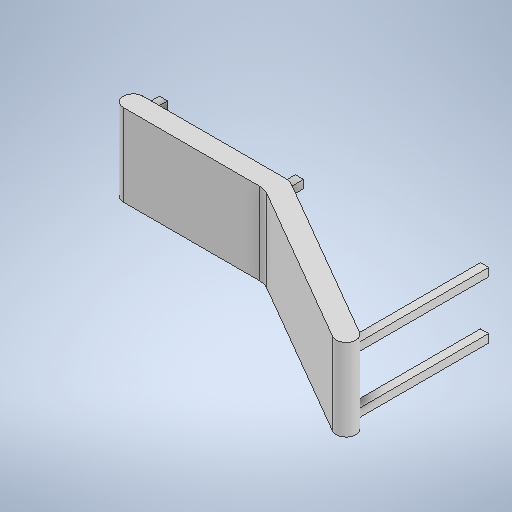
# Autodesk Inventor part: FirstConveyor
Saved by Autodesk Inventor 2025.1 (Build 291241000, 241)
## iProperties
Created: 2025-02-20
Part Number: FirstConveyor
Material: Generic
Document SubType Name: Modeling
Designer: yovan
Density: 1 g/cm^3
Appearance: Default
Author: yovan
Autodesk Inventor part; units mm, degrees
ref_plane "YZ Plane" through (0, 0, 0) normal (1, 0, 0) x (0, 1, 0)
ref_plane "XZ Plane" through (0, 0, 0) normal (0, 1, 0) x (-1, 0, 0)
ref_plane "XY Plane" through (0, 0, 0) normal (0, 0, 1) x (1, 0, 0)
sketch "Sketch1" plane through (0, 0, 0) normal (0, 1, 0) x (-1, 0, 0)
  line L0 (-60, 0) -> (-940, 0)
  line L1 (-891.5776, 120) -> (-60, 120)
  arc A0 (-60, 0) -> (-60, 120) centre (-60, 60) ccw
  line L2 (-60, 0) -> (-90, 0)
  arc A1 (-1909.8969, 691.9019) -> (-1970.1031, 588.0981) centre (-1940, 640) ccw
  line L3 (-1909.8969, 691.9019) -> (-951.7838, 136.1963)
  line L4 (-1970.1031, 588.0981) -> (-970.1031, 8.0981)
  arc A2 (-951.7838, 136.1963) -> (-891.5776, 120) centre (-891.5776, 240) ccw
  arc A3 (-970.1031, 8.0981) -> (-940, 0) centre (-940, 60) ccw
  line L5 (-60, 0) -> (-110, 0)
  line L6 (-110, 0) -> (-110, -100)
  line L7 (-110, -100) -> (-60, -100)
  line L8 (-60, -100) -> (-60, 0)
  line L9 (-940, 0) -> (-890, 0)
  line L10 (-890, 0) -> (-890, -100)
  line L11 (-890, -100) -> (-940, -100)
  line L12 (-940, -100) -> (-940, 0)
  line L13 (-1920.1031, 559.0981) -> (-1920.1031, -199.9999)
  line L14 (-1920.1031, -199.9999) -> (-1970.1031, -199.9999)
  line L15 (-1970.1031, -199.9999) -> (-1970.1031, 588.0981)
  point P0 (0, 0)
  dimension "d9" = 120
  dimension "d10" = 50
  dimension "d11" = 100
  dimension "d12" = 50
  dimension "d13" = 100
  dimension "d16" = 50
  constraints: 32 end point, 8 point on circle, 6 parallel, 4 centre point, 4 horizontal, 2 perpendicular, 2 tangent, 1 point on line
  measures "d9" radius of A2
  measures "d10" distance of L7.end L6.end
  measures "d11" distance of L6.end L5.end
  measures "d12" distance of L10.end L11.end
  measures "d13" distance of L9.end L10.end
  measures "d16" distance of L13.end L14.end
extrude "Extrusion1" add sketch "Sketch1" against normal blind 50 contours L8 L7 L6 L0 | L10 L11 L12 L0 | L4 L13 L14 L15
extrude "Extrusion2" add sketch "Sketch1" against normal blind 450 contours L0 A3 L4 A1 L3 A2 L1 A0
extrude "Extrusion3" add sketch "Sketch1" along normal blind 50 contours L0 A3 L4 A1 L3 A2 L1 A0
sketch "Sketch2" plane through (940, -450, 0) normal (0, 0, -1) x (-1, 0, 0)
  line L0 (880, 400) -> (880, 0) projected
  line L1 (880, 50) -> (830, 50)
  line L2 (830, 50) -> (830, 100)
  line L3 (830, 100) -> (880, 100)
  line L4 (880, 100) -> (880, 50)
  line L5 (0, 400) -> (0, 0) projected
  line L6 (0, 50) -> (50, 50)
  line L7 (50, 50) -> (50, 100)
  line L8 (50, 100) -> (0, 100)
  line L9 (0, 100) -> (0, 50)
  line L10 (-1030.1031, 50) -> (-980.1031, 50)
  line L11 (-980.1031, 50) -> (-980.1031, 100)
  line L12 (-980.1031, 100) -> (-1030.1031, 100)
  line L13 (-1030.1031, 100) -> (-1030.1031, 50)
  point P0 (940, 450)
  dimension "d24" = 50
  dimension "d25" = 50
  dimension "d26" = 50
  dimension "d27" = 50
  dimension "d28" = 50
  dimension "d29" = 50
  constraints: 24 end point, 6 parallel, 3 horizontal, 3 perpendicular, 2 point on line
  measures "d24" distance of L2.end L3.end
  measures "d25" distance of L1.end L2.end
  measures "d26" distance of L8.end L7.end
  measures "d27" distance of L7.end L6.end
  measures "d28" distance of L12.end L11.end
  measures "d29" distance of L11.end L10.end
extrude "Extrusion4" add sketch "Sketch2" along normal blind 100 contours L0 L1 L2 L3 | L8 L7 L6 L5
extrude "Extrusion5" add sketch "Sketch2" along normal blind 200 contours L13 L12 L11 L10
extrude "Extrusion6" add sketch "Sketch2" against normal blind 600 contours L13 L12 L11 L10
body "Solid1"
